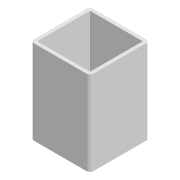
# Autodesk Inventor part: 00_Laser_match_housing
Saved by Autodesk Inventor 2022 (Build 260153000, 153)
## iProperties
Created: 2021-11-18
Part Number: 00_Laser_match_housing
Material: Generic
Document SubType Name: Modeling
Designer: diederichbenedict
Density: 1 g/cm^3
Appearance: Default
Author: diederichbenedict
Autodesk Inventor part; units mm, degrees
ref_plane "YZ Plane" through (0, 0, 0) normal (1, 0, 0) x (0, 1, 0)
ref_plane "XZ Plane" through (0, 0, 0) normal (0, 1, 0) x (-1, 0, 0)
ref_plane "XY Plane" through (0, 0, 0) normal (0, 0, 1) x (1, 0, 0)
sketch "Sketch1" plane through (0, 0, 0) normal (0, 1, 0) x (-1, 0, 0)
  line L0 (-16.95, -16.95) -> (16.95, -16.95)
  line L1 (16.95, -16.95) -> (16.95, 16.95)
  line L2 (16.95, 16.95) -> (-16.95, 16.95)
  line L3 (-16.95, 16.95) -> (-16.95, -16.95)
  line L4 (-16.95, -16.95) -> (16.95, 16.95) construction
  line L5 (16.95, -16.95) -> (-16.95, 16.95) construction
  line L6 (-15, -15) -> (15, -15)
  line L7 (15, -15) -> (15, 15)
  line L8 (15, 15) -> (-15, 15)
  line L9 (-15, 15) -> (-15, -15)
  line L10 (-15, -15) -> (15, 15) construction
  line L11 (15, -15) -> (-15, 15) construction
  point P0 (0, 0)
  dimension "d0" = 33.9
  dimension "d1" = 33.9
  dimension "d2" = 30
  dimension "d3" = 30
  constraints: 24 end point, 4 midpoint, 4 parallel, 2 horizontal, 2 perpendicular
  measures "d0" distance of L2.end L1.end
  measures "d1" distance of L1.end L0.end
  measures "d2" distance of L8.end L7.end
  measures "d3" distance of L7.end L6.end
extrude "Extrusion1" add sketch "Sketch1" along normal blind 48
fillet "Fillet1" radius 2 4 edges at (16.95, 24, 16.95) (16.95, 24, -16.95) (-16.95, 24, -16.95) (-16.95, 24, 16.95)
body "Solid1"
